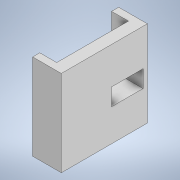
# Autodesk Inventor part: traffic nano
Saved by Autodesk Inventor 2022.1 (Build 261234020, 234B)
## iProperties
Created: 2022-01-09
Part Number: traffic nano
Material: Generic
Document SubType Name: Modeling
Designer: 46734
Density: 1 g/cm^3
Appearance: Default
Author: 46734
Autodesk Inventor part; units mm, degrees
ref_plane "YZ Plane" through (0, 0, 0) normal (1, 0, 0) x (0, 1, 0)
ref_plane "XZ Plane" through (0, 0, 0) normal (0, 1, 0) x (-1, 0, 0)
ref_plane "XY Plane" through (0, 0, 0) normal (0, 0, 1) x (1, 0, 0)
sketch "Sketch1" plane through (0, 0, 0) normal (0, 1, 0) x (-1, 0, 0)
  line L0 (20, 30) -> (-20, 30)
  line L1 (-20, 30) -> (-20, -30)
  line L2 (-20, -30) -> (20, -30)
  line L3 (20, -30) -> (20, 30)
  line L4 (20, 30) -> (-20, -30) construction
  line L5 (-20, 30) -> (20, -30) construction
  point P0 (0, 0)
  dimension "d0" = 40
  dimension "d1" = 60
  constraints: 12 end point, 2 midpoint, 2 parallel, 1 horizontal, 1 perpendicular
  measures "d0" distance of L1.end L2.end
  measures "d1" distance of L2.end L0.start
extrude "Extrusion1" add sketch "Sketch1" along normal blind 60
sketch "Sketch2" plane through (0, 0, 0) normal (0, -1, 0) x (1, 0, 0)
  line L0 (-18, 28) -> (18, 28)
  line L1 (18, 28) -> (18, -28)
  line L2 (18, -28) -> (-18, -28)
  line L3 (-18, -28) -> (-18, 28)
  line L4 (-18, 28) -> (18, -28) construction
  line L5 (18, 28) -> (-18, -28) construction
  line L6 (-20, -30) -> (-20, 30) projected
  line L7 (-20, 30) -> (20, 30) projected
  point P0 (0, 0)
  dimension "d12" = 56
  dimension "d13" = 36
  constraints: 12 end point, 2 midpoint, 2 parallel, 1 horizontal, 1 perpendicular
  measures "d12" distance of L0.end L1.end
  measures "d13" distance of L0.end L0.start
extrude "Extrusion2" cut sketch "Sketch2" against normal blind 20
sketch "Sketch3" plane through (0, 60, 0) normal (0, 1, 0) x (1, 0, 0)
  line L0 (-11.8113, 25.0498) -> (11.8113, 25.0498)
  line L1 (11.8113, 25.0498) -> (11.8113, -25.0498)
  line L2 (11.8113, -25.0498) -> (-11.8113, -25.0498)
  line L3 (-11.8113, -25.0498) -> (-11.8113, 25.0498)
  line L4 (-11.8113, 25.0498) -> (11.8113, -25.0498) construction
  line L5 (11.8113, 25.0498) -> (-11.8113, -25.0498) construction
  point P0 (0, 0)
  dimension "d8" = 50.0996
  dimension "d9" = 23.6226
  constraints: 12 end point, 2 midpoint, 2 parallel, 1 horizontal, 1 perpendicular
  measures "d8" distance of L0.end L1.end
  measures "d9" distance between parallel lines of L3 L1
extrude "Extrusion3" cut sketch "Sketch3" against normal blind 18
sketch "Sketch4" plane through (20, 0, 30) normal (1, 0, 0) x (0, 0, -1)
  line L0 (35, 34.3773) -> (57, 34.3773)
  line L1 (57, 34.3773) -> (57, 22.3773)
  line L2 (57, 22.3773) -> (35, 22.3773)
  line L3 (35, 22.3773) -> (35, 34.3773)
  line L4 (0, 0) -> (0, 60) projected
  point P0 (30, 0)
  point P1 (0, 30)
  dimension "d14" = 22
  dimension "d15" = 12
  dimension "d16" = 35
  constraints: 8 end point, 2 parallel, 1 horizontal, 1 midpoint, 1 perpendicular
  measures "d14" distance of L1.end L2.end
  measures "d15" distance of L0.end L1.end
  measures "d16" distance from line of point (0, 30) L3
extrude "Extrusion4" cut sketch "Sketch4" against normal through all
sketch "Sketch5" plane through (0, 42, 0) normal (0, 1, 0) x (1, 0, 0)
  line L0 (7.446, 22.5061) -> (-3.975, 22.5061)
  line L1 (-3.975, 22.5061) -> (-3.975, 12.3168)
  line L2 (-3.975, 12.3168) -> (7.446, 12.3168)
  line L3 (7.446, 12.3168) -> (7.446, 22.5061)
  point P0 (0, 0)
  constraints: 8 end point, 2 parallel, 1 horizontal, 1 perpendicular
extrude "Extrusion5" cut sketch "Sketch5" against normal through all
sketch "Sketch6" plane through (20, 0, -30) normal (0, 0, -1) x (-1, 0, 0)
  line L0 (40, 0) -> (40, 60) projected
  line L1 (20, 0) -> (40, 0)
  line L2 (40, 0) -> (40, 60)
  line L3 (40, 60) -> (20, 60)
  line L4 (20, 60) -> (20, 0)
  constraints: 8 end point, 2 parallel, 1 horizontal, 1 perpendicular
extrude "Extrusion6" cut sketch "Sketch6" against normal through all
body "Solid1"
